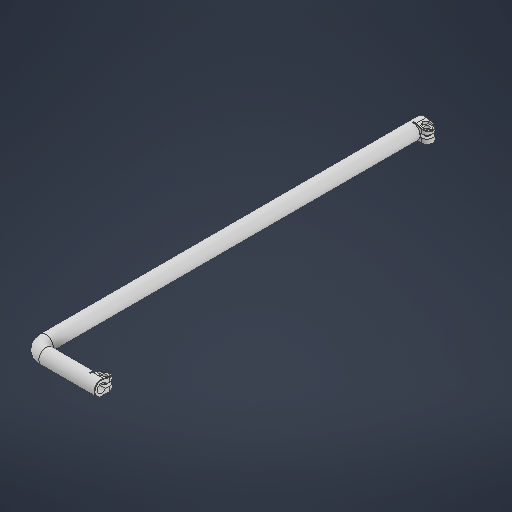
# Autodesk Inventor part: BackpackFrameBottomLeftCorner
Saved by Autodesk Inventor 2026.1 (Build 301233020, 233B)
## iProperties
Created: 2025-10-05
Part Number: BackpackFrameBottomLeftCorner
Material: Generic
Document SubType Name: Modeling
Designer: skybound
Density: 1 g/cm^3
Appearance: Default
Author: skybound
Autodesk Inventor part; units mm, degrees
ref_plane "YZ Plane" through (0, 0, 0) normal (1, 0, 0) x (0, 1, 0)
sketch "Sketch2" plane through (0, 0, 0) normal (0, 1, 0) x (-1, 0, 0)
  line L0 (-48, 0) -> (-8, 0)
  arc A0 (0, -8) -> (-8, 0) centre (-8, -8) ccw
  line L1 (0, -8) -> (0, -280)
  point P0 (0, 0)
  dimension "d3" = 280
  dimension "d4" = 48
  dimension "d5" = 8
  constraints: 4 end point, 2 point on circle, 2 point on line, 2 tangent, 1 centre point, 1 horizontal, 1 vertical
  measures "d3" distance of point (0, 0) L1.end
  measures "d4" distance of L0.start point (0, 0)
  measures "d5" radius of A0
ref_plane "Work Plane1" through (48, 0, 0) normal (-1, 0, 0) x (0, -1, 0)
sketch "Sketch3" plane through (48, 0, 0) normal (-1, 0, 0) x (0, -1, 0)
  circle A0 centre (0, 0) radius 3.25
  circle A1 centre (0, 0) radius 5.25
  line L0 (4.300548, 3.011276) -> (5.25, 1.655319)
  line L1 (5.25, 1.655319) -> (5.25, -1.655319)
  line L2 (5.25, -1.655319) -> (4.300548, -3.011276)
  line L3 (5.25, 0) -> (0, 0) construction
  dimension "d6" = 6.5
  dimension "d7" = 2
  dimension "d8" = 35
  constraints: 8 end point, 3 tangent, 2 centre point, 2 point on circle, 1 coincident, 1 horizontal, 1 midpoint, 1 vertical
  measures "d6" diameter of A0
  measures "d7" radial gap between concentric circles of A0 A1
  measures "d8" angle of L1 L0
sweep "Sweep1" add profiles "Sketch3" path "Sketch2" contours A0 | A1 | L1 L2 A1 | A1 L0 L1
extrude "Extrusion1" cut sketch "Sketch3" along normal blind 40 contours A0
sketch "Sketch4" plane through (0, 0, -280) normal (0, 0, -1) x (-1, 0, 0)
  circle A0 centre (0, 0) radius 3.25
  line L0 (-48, -3.25) -> (-48, 3.25) projected
  line L1 (0, 3.25) -> (0, -3.25) construction
  point P0 (0, 0)
  constraints: 2 end point, 2 point on circle, 1 centre point, 1 coincident, 1 midpoint, 1 parallel, 1 vertical
extrude "Extrusion2" cut sketch "Sketch4" against normal blind 40
sketch "Sketch8" plane through (48, 0, 0) normal (1, 0, 0) x (0, 0, -1)
  line L0 (3.011276, -4.300548) -> (1.655319, -5.25)
  arc A0 (3.011276, -4.300548) -> (-3.011276, -4.300548) centre (0, 0) ccw
  line L1 (1.655319, -5.25) -> (-1.655319, -5.25)
  line L2 (1.655319, -5.25) -> (9.655319, -5.25)
  line L3 (9.655319, -5.25) -> (9.655319, 2.75)
  line L4 (9.655319, 2.75) -> (1.414663, 5.055811)
  dimension "d25" = 8
  dimension "d26" = 8
  constraints: 6 end point, 1 horizontal, 1 perpendicular, 1 point on circle, 1 tangent
  measures "d25" distance of L0.end L2.end
  measures "d26" distance of L2.end L3.end
extrude "Extrusion6" add sketch "Sketch8" against normal blind 8
sketch "Sketch9" plane through (48, -5.25, -9.655319) normal (1, 0, 0) x (0, 0, -1)
  circle A0 centre (-9.655319, 5.25) radius 3.25
  line L0 (-6.916706, 3.5) -> (0, 3.5)
  line L1 (0, 8) -> (0, 0)
  line L2 (-6.493041, 6) -> (0, 6)
  line L3 (-11.310637, 0) -> (0, 0)
  dimension "d29" = 2.5
  dimension "d30" = 3.5
  constraints: 4 end point, 2 point on circle, 2 point on line, 1 horizontal, 1 perpendicular
  measures "d29" distance between parallel lines of L0 L2
  measures "d30" distance between parallel lines of L3 L0
extrude "Extrusion7" cut sketch "Sketch9" against normal up to surface (8 mm away) contours A0 L2 L1 L0
sketch "Sketch10" plane through (8, -5.25, 1.655319) normal (0, -1, 0) x (1, 0, 0)
  line L0 (32, -11.310637) -> (32, -3.310637)
  line L1 (32, -6.905319) -> (0, -6.905319)
  line L2 (32, -3.310637) -> (32, -1.655319)
  line L3 (32, -1.655319) -> (31.6, -1.655319)
  line L4 (31.6, -1.655319) -> (31.6, -6.905319)
  point P0 (-8, -1.655319)
  dimension "d33" = 0.4
  dimension "d34" = 5.25
  constraints: 6 end point, 2 perpendicular, 1 point on line, 1 vertical
  measures "d33" distance of L2.end L3.end
  measures "d34" distance of L3.end L4.end
extrude "Extrusion8" cut sketch "Sketch10" against normal through all
sketch "Sketch11" plane through (8, -5.25, 1.655319) normal (0, -1, 0) x (1, 0, 0)
  line L0 (40, -11.310637) -> (32, -11.310637)
  line L1 (36, -11.310637) -> (36, -7.310637) construction
  circle A0 centre (36, -7.310637) radius 1.7
  point P0 (-8, -1.655319)
  dimension "d37" = 3.4
  dimension "d38" = 4
  constraints: 2 end point, 1 centre point, 1 coincident, 1 midpoint, 1 vertical
  measures "d37" diameter of A0
  measures "d38" distance of L1.start L1.end
hole "Hole1" at (44, -5.25, -5.655319) direction (0, 1, 0) diameter 3.4 end through all counterbore diameter 6.5 counterbore depth 1.5
ref_plane "Work Plane2" through (48, 5.25, 0) normal (0, 1, 0) x (-1, 0, 0)
sketch "Sketch12" plane through (48, 5.25, 0) normal (0, 1, 0) x (-1, 0, 0)
  circle A0 centre (4, -5.655319) radius 1.7
  line L0 (6.9, -3.981003) -> (6.9, -7.329634)
  line L1 (6.9, -7.329634) -> (4, -9.00395)
  line L2 (4, -9.00395) -> (1.1, -7.329634)
  line L3 (1.1, -7.329634) -> (1.1, -3.981003)
  line L4 (1.1, -3.981003) -> (4, -2.306687)
  line L5 (4, -2.306687) -> (6.9, -3.981003)
  point P0 (48, 0)
  dimension "d47" = 5.8
  constraints: 12 end point, 1 coincident, 1 vertical, 13 other
  measures "d47" distance between parallel lines of L3 L0
extrude "Extrusion9" cut sketch "Sketch12" against normal blind 2.5
sketch "Sketch13" plane through (0, 0, -280) normal (0, 0, -1) x (-1, 0, 0)
  line L0 (-3.011276, -4.300548) -> (-1.655319, -5.25)
  line L1 (-1.655319, -5.25) -> (-9.655319, -5.25)
  line L2 (-8, -5.25) -> (-1.655319, -5.25)
  line L3 (-9.655319, -5.25) -> (-9.655319, 2.75)
  line L4 (-9.655319, 2.75) -> (-1.414663, 5.055811)
  arc A0 (3.011276, -4.300548) -> (-3.011276, -4.300548) centre (0, 0) ccw
  line L5 (-48, -5.25) -> (-48, 2.75)
  point P0 (0, 0)
  dimension "d50" = 8
  constraints: 6 end point, 1 collinear, 1 parallel, 1 perpendicular, 1 point on circle, 1 tangent
  measures "d50" distance of L0.end L1.end
extrude "Extrusion10" add sketch "Sketch13" against normal blind 8
sketch "Sketch14" plane through (9.655319, -5.25, -280) normal (0, 0, -1) x (-1, 0, 0)
  line L0 (0, 0) -> (0, 8)
  line L1 (0, 6) -> (6.493041, 6)
  circle A0 centre (9.655319, 5.25) radius 3.25
  line L2 (6.916706, 3.5) -> (0, 3.5)
  line L3 (0, 0) -> (11.310637, 0)
  line L4 (-30.344681, 3.5) -> (-38.344681, 3.5)
  line L5 (-38.344681, 6) -> (-30.344681, 6)
  point P0 (9.655319, 5.25)
  point P1 (0, 3.5)
  constraints: 4 end point, 2 collinear, 2 horizontal, 2 point on circle, 1 point on line
extrude "Extrusion11" cut sketch "Sketch14" against normal up to surface (8 mm away) contours L0 L1 A0 L2
sketch "Sketch15" plane through (8, -5.25, 1.655319) normal (0, -1, 0) x (1, 0, 0)
  line L0 (-6.344681, -273.655319) -> (1.655319, -273.655319)
  line L1 (1.655319, -273.655319) -> (-8, -273.655319)
  line L2 (-8, -273.655319) -> (-8, -273.255319)
  line L3 (-8, -273.255319) -> (1.655319, -273.255319)
  line L4 (1.655319, -273.255319) -> (1.655319, -273.655319)
  line L5 (32, -1.655319) -> (32, -11.310637)
  line L6 (31.6, -1.655319) -> (32, -1.655319)
  point P0 (-8, -1.655319)
  constraints: 8 end point, 5 perpendicular, 1 horizontal
extrude "Extrusion12" cut sketch "Sketch15" against normal through all
sketch "Sketch16" plane through (8, -5.25, 1.655319) normal (0, -1, 0) x (1, 0, 0)
  line L0 (1.655319, -281.655319) -> (1.655319, -273.655319)
  line L1 (1.655319, -277.655319) -> (-2.344681, -277.655319) construction
  circle A0 centre (-2.344681, -277.655319) radius 1.7
  point P0 (-8, -1.655319)
  dimension "d59" = 3.4
  dimension "d60" = 4
  constraints: 2 end point, 1 centre point, 1 coincident, 1 horizontal, 1 midpoint
  measures "d59" diameter of A0
  measures "d60" distance of L1.start L1.end
hole "Hole2" at (5.655319, -5.25, -276) direction (0, 1, 0) diameter 3.4 end through all counterbore diameter 6.5 counterbore depth 1.5
sketch "Sketch17" plane through (48, 5.25, 0) normal (0, 1, 0) x (-1, 0, 0)
  circle A0 centre (42.344681, -276) radius 1.7
  line L0 (44.018997, -273.1) -> (45.693313, -276)
  line L1 (45.693313, -276) -> (44.018997, -278.9)
  line L2 (44.018997, -278.9) -> (40.670366, -278.9)
  line L3 (40.670366, -278.9) -> (38.99605, -276)
  line L4 (38.99605, -276) -> (40.670366, -273.1)
  line L5 (40.670366, -273.1) -> (44.018997, -273.1)
  line L6 (1.1, -7.329634) -> (1.1, -3.981003)
  point P0 (48, 0)
  constraints: 12 end point, 1 coincident, 1 horizontal, 1 perpendicular, 13 other
extrude "Extrusion13" cut sketch "Sketch17" against normal blind 2.5 contours A0 | L0 L1 L2 L3 L4 L5
fillet "Fillet2" radius 0.2 8 edges at (39.6, -4.25, 0) (39.6, 4.25, 0) (40, -4.25, 0) (40, 4.25, 0) (0, -4.25, -272) (0, 4.25, -272) (0, -4.25, -271.6) (0, 4.25, -271.6)
fillet "Fillet3" radius 4 8 edges at (9.6553, -3.5, -272) (9.6553, 1.75, -272) (9.6553, 1.75, -280) (9.6553, -3.5, -280) (48, 1.75, -9.6553) (40, 1.75, -9.6553) (40, -3.5, -9.6553) (48, -3.5, -9.6553)
fillet "Fillet4" radius 0.25 49 edges at (3.535, 4.4625, -280) (8.4838, 3.0778, -273.1715) (3.535, 4.4625, -272) (0.8129, 5.1867, -272) (0, -5.25, -271.9) (0, -5.25, -271.7) (39.9, -5.25, 0) (39.7, -5.25, 0) (0.0586, -5.25, -271.9414) (0.0586, -5.25, -271.6586) (39.9414, -5.25, -0.0586) (39.6586, -5.25, -0.0586) (0.1, 5.249, -272) (0, 5.25, -271.7) (0, 5.25, -271.9) (0.1, 5.249, -271.6) (40, 5.249, -0.1) (39.9, 5.25, 0) (39.7, 5.25, 0) (39.6, 5.249, -0.1) (0.058, 5.2497, -271.6592) (39.6592, 5.2497, -0.058) (0.058, 5.2497, -271.9408) (39.9408, 5.2497, -0.058) (5.0362, 1.483, -271.6) (2.3333, -4.7753, -271.6) (-2.3333, -4.7753, -280) (-4.7458, 2.245, -280) (8.4838, -5.25, -278.8285) (8.4838, -5.25, -273.1715) (2.9277, -5.25, -272) (0.1, -5.25, -271.6) (0.9277, -5.25, -271.6) (2, -5.25, -280) (48, 4.4625, -3.535) (48, 2.245, 4.7458) (48, -4.7753, 2.3333) (40, 4.4625, -3.535) (40, 5.1867, -0.8129) (39.6, 1.483, -5.0362) (39.6, -4.7753, -2.3333) (44, 2.75, -9.6553) (46.8285, 3.0778, -8.4838) (40, -5.25, -2.9277) (39.6, -5.25, -0.1) (39.6, -5.25, -0.9277) (48, -5.25, -2.0001) (46.8285, -5.25, -8.4838) (41.1715, -5.25, -8.4838)
chamfer "Chamfer1" distance 0.25 angle 45 10 edges at (-1.6553, -5.25, -143.875) (1.1727, -5.25, -1.1727) (27.875, -5.25, 1.6553) (-1.6322, -5.1768, -279.9268) (47.9268, -5.1768, 1.6322) (1.6553, -5.25, -139.675) (3.5136, -5.25, -3.5136) (23.675, -5.25, -1.6553) (1.6322, -5.1768, -271.5268) (39.5268, -5.1768, -1.6322)
body "Solid1"
